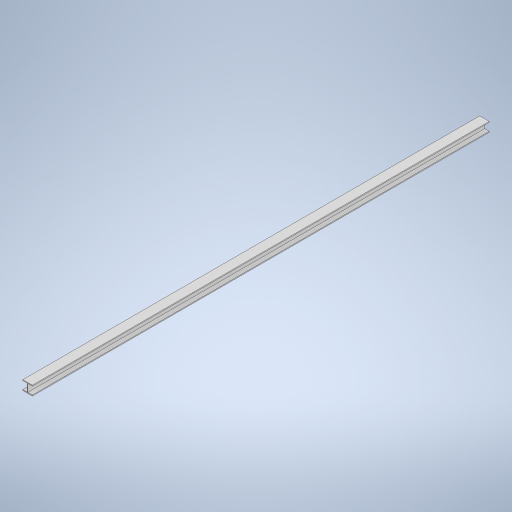
# Autodesk Inventor part: SpaceX Track
Saved by Autodesk Inventor 2023 (Build 270158000, 158)
## iProperties
Created: 2022-03-31
Part Number: SpaceX Track
Material: Generic
Document SubType Name: Modeling
Designer: Zain Ali
Density: 1 g/cm^3
Appearance: Default
Author: Zain Ali
Autodesk Inventor part; units mm, degrees
ref_plane "YZ Plane" through (0, 0, 0) normal (1, 0, 0) x (0, 1, 0)
ref_plane "XZ Plane" through (0, 0, 0) normal (0, 1, 0) x (-1, 0, 0)
ref_plane "XY Plane" through (0, 0, 0) normal (0, 0, 1) x (1, 0, 0)
sketch "Sketch2" plane through (0, 0, 0) normal (0, 0, 1) x (1, 0, 0)
  line L0 (0, 0) -> (127, 0)
  line L1 (127, 0) -> (127, -12.7)
  line L2 (127, -12.7) -> (67.31, -12.7)
  line L3 (67.31, -12.7) -> (67.31, -114.3)
  line L4 (67.31, -114.3) -> (127, -114.3)
  line L5 (127, -114.3) -> (127, -127)
  line L6 (127, -127) -> (0, -127)
  line L7 (0, -127) -> (0, -114.3)
  line L8 (0, -114.3) -> (59.69, -114.3)
  line L9 (59.69, -114.3) -> (59.69, -12.7)
  line L10 (59.69, -12.7) -> (0, -12.7)
  line L11 (0, 0) -> (0, -12.7)
  dimension "d11" = 12.7
  dimension "d12" = 127
  dimension "d13" = 127
  dimension "d14" = 12.7
  dimension "d15" = 59.69
  dimension "d16" = 59.69
  constraints: 24 end point, 8 perpendicular, 7 point on line, 1 horizontal
  measures "d11" distance of L0.end L1.end
  measures "d12" distance of L0.start L0.end
  measures "d13" distance between parallel lines of L6 L0
  measures "d14" distance of L6.end L7.end
  measures "d15" distance of L1.end L2.end
  measures "d16" distance of L9.end L10.end
extrude "Extrusion1" add sketch "Sketch2" along normal blind 6096
body "Solid2"
